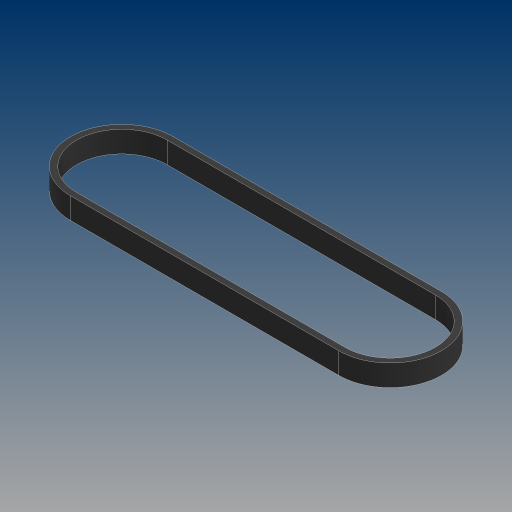
# Autodesk Inventor part: SHOT_1_014_Belt3
Saved by Autodesk Inventor 2024.3 (Build 283343000, 343)
## iProperties
Created: 2024-08-09
Part Number: SHOT_1_014_Belt3
Material: Rubber, Silicone
Document SubType Name: Modeling
Designer: Kenji
Density: 1.25 g/cm^3
Appearance: Rubber - Black
Author: Kenji
Autodesk Inventor part; units mm, degrees
ref_plane "YZ Plane" through (0, 0, 0) normal (1, 0, 0) x (0, 1, 0)
ref_plane "XZ Plane" through (0, 0, 0) normal (0, 1, 0) x (-1, 0, 0)
ref_plane "XY Plane" through (0, 0, 0) normal (0, 0, 1) x (1, 0, 0)
sketch "Sketch1" plane through (0, 0, 0) normal (0, 1, 0) x (-1, 0, 0)
  circle A0 centre (0, 0) radius 19.1008 construction
  line L0 (0, 0) -> (113.1223, 0) construction
  circle A1 centre (113.1223, 0) radius 19.1008 construction
  line L1 (113.1223, 19.1008) -> (0, 19.1008)
  line L2 (113.1223, -19.1008) -> (0, -19.1008)
  arc A2 (113.1223, -19.1008) -> (113.1223, 19.1008) centre (113.1223, 0) ccw
  arc A3 (0, 19.1008) -> (0, -19.1008) centre (0, 0) ccw
  line L3 (0, 21.6408) -> (113.1223, 21.6408)
  arc A4 (113.1223, -21.6408) -> (113.1223, 21.6408) centre (113.1223, 0) ccw
  line L4 (113.1223, -21.6408) -> (0, -21.6408)
  arc A5 (0, 21.6408) -> (0, -21.6408) centre (0, 0) ccw
  dimension "d0" = 38.2016
  dimension "d1" = 38.2016
  dimension "d2" = 113.1223
  dimension "d3" = 2.54
  constraints: 12 point on circle, 10 end point, 6 centre point, 5 tangent, 2 coincident, 2 horizontal, 2 parallel, 3 other
  measures "d0" diameter of A0
  measures "d1" diameter of A1
  measures "d2" distance of L0.start L0.end
  measures "d3" distance between parallel lines of L1 L3
extrude "Extrusion1" add sketch "Sketch1" along normal blind 9
body "Solid1"
